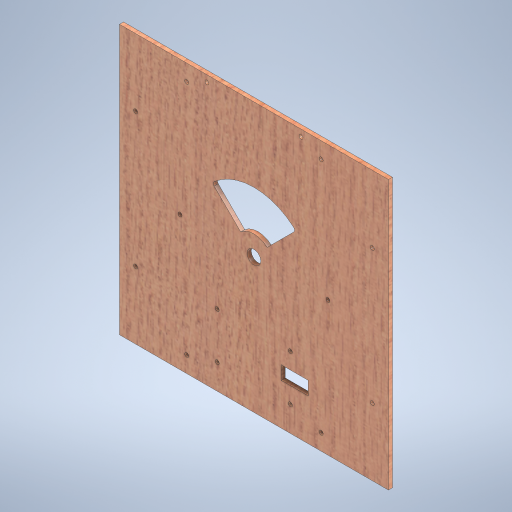
# Autodesk Inventor part: Soporte_Dosificador
Saved by Autodesk Inventor 2024 (Build 280153000, 153)
## iProperties
Created: 2024-07-16
Part Number: Soporte_Dosificador
Material: Genérico
Document SubType Name: Modeling
Designer: sergi
Density: 1 g/cm^3
Appearance: Valor por defecto
Author: sergi
Autodesk Inventor part; units mm, degrees
ref_plane "YZ Plane" through (0, 0, 0) normal (1, 0, 0) x (0, 1, 0)
ref_plane "XZ Plane" through (0, 0, 0) normal (0, 1, 0) x (-1, 0, 0)
ref_plane "XY Plane" through (0, 0, 0) normal (0, 0, 1) x (1, 0, 0)
sketch "Boceto1" plane through (0, 0, 0) normal (0, 0, 1) x (1, 0, 0)
  line L0 (-103, 100) -> (-103, -103)
  line L1 (-103, 100) -> (-100, 100)
  line L2 (-100, -103) -> (-100, 100)
  line L3 (-103, -103) -> (-100, -103)
  line L4 (100, 103) -> (-103, 103)
  line L5 (100, 103) -> (100, 100)
  line L6 (-103, 100) -> (100, 100)
  line L7 (-103, 103) -> (-103, 100)
  line L8 (-100, -103) -> (103, -103)
  line L9 (-100, -103) -> (-100, -100)
  line L10 (103, -100) -> (-100, -100)
  line L11 (103, -103) -> (103, -100)
  line L12 (100, -98) -> (100, 100)
  line L13 (100, 100) -> (98, 100)
  circle A0 centre (0, 0) radius 3.9
  circle A1 centre (0, 0) radius 8
  circle A2 centre (0, 0) radius 3.9
  circle A3 centre (0, 0) radius 4
  line L14 (103, 100) -> (103, -103)
  line L15 (100, -103) -> (100, 100)
  line L16 (103, -103) -> (100, -103)
  circle A4 centre (0, 0) radius 5.1
  line L17 (103, 100) -> (100, 100)
  point P0 (100, -100)
extrude "Extrusión1" add sketch "Boceto1" along normal blind 3 contours L6 L12 L15 L10 L2 | A1
sketch "Boceto2" plane through (0, 0, 3) normal (0, 0, 1) x (1, 0, 0)
  circle A0 centre (0, 0) radius 45
  line L0 (-4.4142, 5.8284) -> (-29.6244, 31.0386)
  arc A1 (-3.1395, 44.8903) -> (-29.5223, 33.9623) centre (0, 0) ccw
  line L1 (29.6244, 31.0386) -> (4.4142, 5.8284)
  arc A2 (29.5223, 33.9623) -> (3.1395, 44.8903) centre (0, 0) ccw
  arc A3 (-29.5223, 33.9623) -> (-29.6244, 31.0386) centre (-28.2102, 32.4528) ccw
  arc A4 (29.6244, 31.0386) -> (29.5223, 33.9623) centre (28.2102, 32.4528) ccw
  circle A5 centre (0, 0) radius 8
  circle A6 centre (0, 0) radius 8
  arc A7 (10.4625, 10.7488) -> (-10.4625, 10.7488) centre (0, 0) ccw projected
  point P0 (36.7643, -25.9497)
  point P1 (-36.7643, -25.9497)
  point P2 (-4.9054, 6.3196)
  point P3 (4.9054, 6.3196)
  point P4 (-9.8759, 11.2901)
  point P5 (9.8759, 11.2901)
  constraints: 8 point on circle, 7 centre point, 4 end point
extrude "Extrusión2" cut sketch "Boceto2" against normal blind 3 contours A4 L1 A7 L0 A3 A0
sketch "Boceto4" plane through (0, 0, 3) normal (0, 0, 1) x (1, 0, 0)
  circle A0 centre (0, 0) radius 55
  circle A1 centre (0, 0) radius 5.1 projected
  line L0 (0, 0) -> (55, 0)
  circle A2 centre (55, 0) radius 1.5
  circle A3 centre (-55, 0) radius 1.5
  dimension "d14" = 55
  dimension "d15" = 3
  dimension "d16" = 3
  constraints: 2 centre point, 2 end point, 1 coincident, 1 horizontal, 1 horizontal alignment, 2 other
  measures "d14" distance of L0.start L0.end
  measures "d15" diameter of A2
  measures "d16" diameter of A3
hole "Agujero2" at (55, 0, 3) at (-55, 0, 3) direction (0, 0, -1) diameter 3 depth 4
sketch "Boceto5" plane through (0, 0, 0) normal (0, 0, -1) x (-1, 0, 0)
  circle A0 centre (88, -50) radius 2.1 projected
  circle A1 centre (50, -88) radius 2.1 projected
  circle A2 centre (-50, -88) radius 2.1 projected
  circle A3 centre (-88, -50) radius 2.1 projected
  circle A4 centre (-88, 50) radius 2.1 projected
  circle A5 centre (-50, 88) radius 2.1 projected
  circle A6 centre (50, 88) radius 2.1 projected
  circle A7 centre (88, 50) radius 2.1 projected
  point P0 (0, 0)
hole "Agujero3" at (-88, -50, 0) at (-88, 50, 0) at (-50, 88, 0) at (50, 88, 0) at (88, 50, 0) at (88, -50, 0) at (50, -88, 0) at (-50, -88, 0) direction (0, 0, 1) diameter 3 depth 4
sketch "Boceto6" plane through (0, 0, 3) normal (0, 0, 1) x (1, 0, 0)
  line L0 (20.3165, -69.168) -> (31.0665, -69.168) projected
  line L1 (20.3165, -74.518) -> (20.3165, -69.168) projected
  line L2 (-20.5835, -74.518) -> (20.3165, -74.518) projected
  line L3 (-20.5835, -53.818) -> (-20.5835, -74.518) projected
  line L4 (20.3165, -53.818) -> (-20.5835, -53.818) projected
  line L5 (20.3165, -59.168) -> (20.3165, -53.818) projected
  line L6 (31.0665, -59.168) -> (20.3165, -59.168) projected
  line L7 (31.0665, -43.068) -> (31.0665, -59.168) projected
  line L8 (23.0665, -43.068) -> (31.0665, -43.068) projected
  line L9 (-15.3335, -51.068) -> (15.0665, -51.068) projected
  line L10 (-31.3335, -43.068) -> (-23.3335, -43.068) projected
  line L11 (-31.3335, -85.268) -> (-31.3335, -43.068) projected
  line L12 (-23.3335, -85.268) -> (-31.3335, -85.268) projected
  line L13 (15.0665, -77.268) -> (-15.3335, -77.268) projected
  line L14 (31.0665, -85.268) -> (23.0665, -85.268) projected
  line L15 (31.0665, -69.168) -> (31.0665, -85.268) projected
  circle A0 centre (27.0665, -81.268) radius 2.1 projected
  circle A1 centre (-27.3335, -81.268) radius 2.1 projected
  circle A2 centre (27.0665, -47.068) radius 2.1 projected
  circle A3 centre (-27.3335, -47.068) radius 2.1 projected
  arc A4 (15.0665, -51.068) -> (23.0665, -43.068) centre (15.0665, -43.068) ccw projected
  arc A5 (-23.3335, -43.068) -> (-15.3335, -51.068) centre (-15.3335, -43.068) ccw projected
  arc A6 (-15.3335, -77.268) -> (-23.3335, -85.268) centre (-15.3335, -85.268) ccw projected
  arc A7 (23.0665, -85.268) -> (15.0665, -77.268) centre (15.0665, -85.268) ccw projected
  point P0 (0, 0)
hole "Agujero4" at (27.0665, -81.268, 3) at (27.0665, -47.068, 3) at (-27.3335, -47.068, 3) at (-27.3335, -81.268, 3) direction (0, 0, -1) diameter 3 depth 15
sketch "Boceto7" plane through (0, 0, 0) normal (0, 0, -1) x (-1, 0, 0)
  circle A0 centre (35, 95) radius 2.1 projected
  circle A1 centre (-35, 95) radius 2.1 projected
  circle A2 centre (35, 95) radius 1.5
  point P0 (0, 0)
  dimension "d38" = 3
  constraints: 1 centre point, 1 coincident
  measures "d38" diameter of A2
hole "Agujero5" at (-35, 95, 0) at (35, 95, 0) direction (0, 0, 1) diameter 3 depth 15
sketch "Boceto8" plane through (0, 0, 0) normal (0, 0, -1) x (-1, 0, 0)
  arc A0 (-15.0665, -77.268) -> (-23.0665, -85.268) centre (-15.0665, -85.268) ccw projected
  line L0 (-31.0665, -85.268) -> (-23.0665, -85.268) projected
  line L1 (-31.0665, -69.168) -> (-31.0665, -85.268) projected
  line L2 (-31.0665, -43.068) -> (-31.0665, -59.168) projected
  line L3 (-31.0665, -59.168) -> (-20.3165, -59.168) projected
  line L4 (-20.3165, -69.168) -> (-31.0665, -69.168) projected
  line L5 (-20.0665, -54.068) -> (-20.0665, -74.268) projected
  line L6 (-23.0665, -43.068) -> (-31.0665, -43.068) projected
  line L7 (-20.3165, -69.168) -> (-40.3165, -69.168)
  line L8 (-40.3165, -69.168) -> (-40.3165, -59.168)
  line L9 (-40.3165, -59.168) -> (-20.3165, -59.168)
  line L10 (-20.3165, -59.168) -> (-20.3165, -69.168)
  point P0 (0, 0)
  dimension "d46" = 20
  dimension "d47" = 10
  constraints: 8 end point, 2 parallel, 1 horizontal, 1 perpendicular
  measures "d46" distance of L8.end L9.end
  measures "d47" distance of L7.end L8.end
extrude "Extrusión3" cut sketch "Boceto8" against normal blind 10
